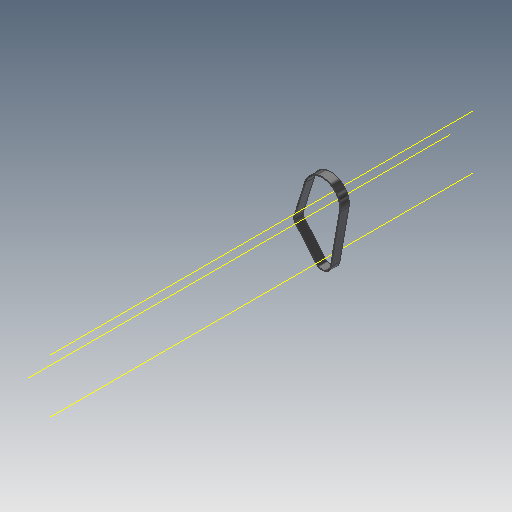
# Autodesk Inventor part: Synchronous Belt
Saved by Autodesk Inventor 2018 (Build 220112000, 112)
## iProperties
Created: 2019-09-22
Part Number: Synchronous Belt
Material: Rubber
Document SubType Name: Modeling
Designer: Clevo
Density: 1 g/cm^3
Appearance: Rubber - Black - Version 1.1
CustomPartVersion: 1
Author: Clevo
Autodesk Inventor part; units mm, degrees
sketch "Sketch Path" plane through (0, 0, 0) normal (0, 0, 1) x (1, 0, 0)
  arc A0 (-4.5858, -3.8198) -> (5.8803, -1.0214) centre (0, 0) ccw
  arc A1 (-19.2993, 16.6817) -> (-18.5572, 12.9535) centre (-15.5, 15.5) ccw
  arc A2 (12.1525, 35.0891) -> (-11.7779, 40.8634) centre (0, 37.2) ccw
  line L0 (12.1525, 35.0891) -> (5.8803, -1.0214)
  line L1 (-4.5858, -3.8198) -> (-18.5572, 12.9535)
  line L2 (-19.2993, 16.6817) -> (-11.7779, 40.8634)
  constraints: 6 end point, 6 point on circle, 3 centre point
ref_plane "Cross Section Plane" through (5.8803, -1.0214, 0) normal (0.1711, 0.9852, 0) x (0, 0, 1)
ref_plane "Work Plane2" through (0, 0, 0) normal (-1, 0, 0) x (0, 0, 1)
ref_plane "Work Plane3" through (-15.5, 15.5, 0) normal (0.2665, -0.9638, 0) x (0, 0, 1)
ref_plane "Work Plane4" through (0, 37.2, 0) normal (-0.4762, -0.8793, 0) x (0, 0, 1)
sketch "Cross Section" plane through (5.8803, -1.0214, 0) normal (0.1711, 0.9852, 0) x (0, 0, 1)
  line L0 (-3, 0.3) -> (3, 0.3)
  line L1 (3, 0.3) -> (3, -0.3)
  line L2 (3, -0.3) -> (-3, -0.3)
  line L3 (-3, -0.3) -> (-3, 0.3)
  line L4 (-3, 0) -> (3, 0) construction
  point P0 (0, 0)
  point P1 (0, 0)
  dimension "d0" = 6
  dimension "d4" = 0.3
  dimension "d5" = 0.3
  constraints: 10 end point, 3 midpoint, 2 parallel, 1 coincident, 1 horizontal, 1 perpendicular, 1 other
  measures "d0" distance between parallel lines of L1 L3
  measures "d4" distance between parallel lines of L2 L4
  measures "d5" distance between parallel lines of L4 L0
sweep "Belt" add profiles "Cross Section" path "Sketch Path"
equation "\"d0\" = da_B"
equation "\"d4\" = da_a"
equation "\"d5\" = da_a2"
equation "\"da_B\" = 6"
equation "\"da_pb\" = 2.5"
equation "\"da_L\" = 138.49893"
equation "\"da_a\" = 0.3"
equation "\"da_S\" = 1.5"
equation "\"da_Beta\" = 20deg"
equation "\"da_Ht\" = 0.7"
equation "\"da_H\" = 1.3"
equation "\"da_a2\" = 0.3"
body "Solid1"
